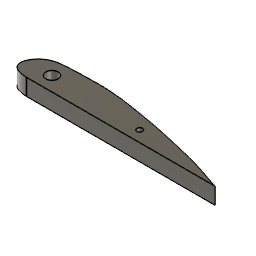
Final_wing_airfoil (Autodesk Fusion 360 design; units mm, degrees)
part number: 2026-06-04-21-35-40-415
Autodesk Fusion 360 part; units mm, degrees
sketch "Sketch4" plane through (0, 0, 0) normal (0, 0, 1) x (1, 0, 0)
  line L0 (0, 0) -> (170, 0)
  spline S0 degree 5 poles (0, 0) (-1.0849, 0.0464) (-3.1503, 0.1925) (-5.9354, 0.5718) (-9.0226, 1.3979) (-11.8442, 2.954) (-13.6498, 5.0011) (-14.4838, 7.4736) (-14.4224, 10.2606) (-13.5809, 13.196) (-12.0967, 16.0888) (-10.1119, 18.7545) (-7.7579, 21.0432) (-5.1347, 22.8761) (-2.3067, 24.2534) (0.6848, 25.2259) (3.812, 25.8759) (7.0515, 26.2956) (10.3717, 26.5634) (13.7341, 26.7374) (17.1006, 26.8598) (20.439, 26.9582) (23.7292, 27.0478) (26.9705, 27.1331) (30.1812, 27.2106) (33.3901, 27.2703) (36.6306, 27.299) (39.9337, 27.2817) (43.3207, 27.2048) (46.8009, 27.0568) (50.374, 26.83) (54.031, 26.5202) (57.7563, 26.1285) (61.5286, 25.6616) (65.3228, 25.1325) (69.1124, 24.5579) (72.8714, 23.9554) (76.5773, 23.3414) (80.2131, 22.7282) (83.7698, 22.1212) (87.2479, 21.5181) (90.6543, 20.9118) (94.0006, 20.2928) (97.3006, 19.6527) (100.5683, 18.9858) (103.8154, 18.2927) (107.052, 17.5781) (110.287, 16.8481) (113.5282, 16.1086) (116.7835, 15.3631) (120.0609, 14.6099) (123.3662, 13.8441) (126.7004, 13.0591) (130.0569, 12.2492) (133.4187, 11.4112) (136.7546, 10.5466) (140.0239, 9.6614) (143.1855, 8.7638) (146.2069, 7.8626) (149.0715, 6.9653) (151.7897, 6.0761) (154.3965, 5.1957) (156.9385, 4.3227) (159.4649, 3.4547) (162.0152, 2.5893) (164.6121, 1.7255) (166.7363, 1.035) (168.3573, 0.5174) (169.4504, 0.1724) (170, 0) knots 0 0 0 0 0 0 0.01538462 0.03076923 0.04615385 0.06153846 0.07692308 0.09230769 0.10769231 0.12307692 0.13846154 0.15384615 0.16923077 0.18461538 0.2 0.21538462 0.23076923 0.24615385 0.26153846 0.27692308 0.29230769 0.30769231 0.32307692 0.33846154 0.35384615 0.36923077 0.38461538 0.4 0.41538462 0.43076923 0.44615385 0.46153846 0.47692308 0.49230769 0.50769231 0.52307692 0.53846154 0.55384615 0.56923077 0.58461538 0.6 0.61538462 0.63076923 0.64615385 0.66153846 0.67692308 0.69230769 0.70769231 0.72307692 0.73846154 0.75384615 0.76923077 0.78461538 0.8 0.81538462 0.83076923 0.84615385 0.86153846 0.87692308 0.89230769 0.90769231 0.92307692 0.93846154 0.95384615 0.96923077 0.98461538 1 1 1 1 1 1
  circle A0 centre (10, 13) radius 5.5
  circle A1 centre (92, 10) radius 2.5
  point P0 (-14.2492, 7.4805)
  point P1 (-8.765, 19.9723)
  point P2 (5, 26)
  point P3 (22, 27)
  point P4 (38.1553, 27.2846)
  point P5 (57.3609, 26.1559)
  point P6 (79.0836, 22.9175)
  point P7 (97.421, 19.6205)
  point P8 (114, 16)
  point P9 (131.2804, 11.9404)
  point P10 (147.4476, 7.4686)
  point P11 (158.799, 3.6848)
  dimension "d5" = 170
  dimension "d7" = 11
  dimension "d8" = 5
  constraint coincident L0.start S0.start
  constraint horizontal L0
  measures "d5" distance of L0.start L0.end
  measures "d7" diameter of A0
  measures "d8" diameter of A1
extrude "Extrude3" add sketch "Sketch4" along normal mid plane 40
extrude "Extrude9" cut 1 faces at (50.6476, 14.9409, -20) along direction (0, 0, 1) blind 10
extrude "Extrude14" cut 1 faces at (50.6476, 14.9409, -10) along direction (0, 0, 1) blind 15
